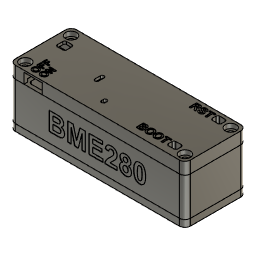
T-Go Energy Thicc v13 (Autodesk Fusion 360 design; units mm, degrees)
Autodesk Fusion 360 part; units mm, degrees
note: some values were not read from the file. Chosen so that the rebuilt part matches the saved one: which face or edge a step refers to; the layout of a text. Set by a fixed rule: which sketch regions a step uses.
(part 1 of 2)
sketch "Sketch1" plane through (0, 0, 0) normal (0, 0, 1) x (1, 0, 0)
  line L0 (0, 0) -> (91.19, 0)
  line L1 (91.19, 0) -> (91.19, -29)
  line L2 (91.19, -29) -> (0, -29)
  line L3 (0, -29) -> (0, 0)
  line L4 (89.22, -2) -> (89.22, -27) construction
  line L5 (89.22, -27) -> (1.97, -27) construction
  line L6 (1.97, -27) -> (1.97, -2) construction
  line L7 (45.595, 0) -> (45.595, -29) construction
  line L8 (0, -14.5) -> (91.19, -14.5) construction
  circle A0 centre (1.97, -2) radius 1.5
  circle A1 centre (89.22, -2) radius 1.5
  circle A2 centre (89.22, -27) radius 1.5
  circle A3 centre (1.97, -27) radius 1.5
  line L9 (7, 2) -> (15, 2)
  line L10 (15, 2) -> (15, -5)
  line L11 (15, -5) -> (7, -5)
  line L12 (7, -5) -> (7, 2)
  line L13 (3.5, -7) -> (6.5, -7)
  line L14 (6.5, -7) -> (6.5, -10)
  line L15 (6.5, -10) -> (3.5, -10)
  line L16 (3.5, -10) -> (3.5, -7)
  line L17 (6, -25.5) -> (15, -25.5)
  line L18 (15, -25.5) -> (15, -29.5)
  line L19 (15, -29.5) -> (6, -29.5)
  line L20 (6, -29.5) -> (6, -25.5)
  line L21 (9, -29.5) -> (11, -29.5)
  line L22 (11, -29.5) -> (11, -31.5)
  line L23 (11, -31.5) -> (9, -31.5)
  line L24 (9, -31.5) -> (9, -29.5)
  line L25 (80.19, 0) -> (84.19, 0)
  line L26 (84.19, 0) -> (84.19, -3)
  line L27 (84.19, -3) -> (80.19, -3)
  line L28 (80.19, -3) -> (80.19, 0)
  line L29 (80.19, -24) -> (84.19, -24)
  line L30 (84.19, -24) -> (84.19, -27)
  line L31 (84.19, -27) -> (80.19, -27)
  line L32 (80.19, -27) -> (80.19, -24)
  line L33 (29, -17) -> (31, -17)
  line L34 (31, -17) -> (31, -12)
  line L35 (31, -12) -> (29, -12)
  line L36 (29, -12) -> (29, -17)
  line L37 (41, -25.4) -> (43, -25.4)
  line L38 (43, -25.4) -> (43, -22.4)
  line L39 (43, -22.4) -> (41, -22.4)
  line L40 (41, -22.4) -> (41, -25.4)
  line L41 (1.97, -2) -> (89.22, -2) construction
  dimension "d1" = 91.19
  dimension "d2" = 29
  dimension "d3" = 3
  dimension "d4" = 84.25
  dimension "d5" = 22
  dimension "d6" = 2
  dimension "d7" = 7
  dimension "d8" = 5
  dimension "d9" = 8
  dimension "d10" = 3.5
  dimension "d11" = 7
  dimension "d12" = 3
  dimension "d13" = 3
  dimension "d14" = 6
  dimension "d15" = 9
  dimension "d16" = 0.5
  dimension "d17" = 9
  dimension "d18" = 11
  dimension "d19" = 2.5
  dimension "d20" = 3.5
  dimension "d21" = 7
  dimension "d22" = 4
  dimension "d23" = 3
  dimension "d24" = 2
  dimension "d84" = 29
  dimension "d85" = 12
  dimension "d87" = 12
  dimension "d88" = 2
  dimension "d110" = 2
  dimension "d111" = 3
  dimension "d126" = 3.6
  dimension "d127" = 41
  constraint horizontal L0
  constraint vertical L1
  constraint horizontal L2
  constraint vertical L3
  constraint coincident L0.start L3.end
  constraint vertical L4
  constraint horizontal L5
  constraint vertical L6
  constraint midpoint L0 L7.start
  constraint midpoint L2 L7.end
  constraint midpoint L3 L8.start
  constraint midpoint L1 L8.end
  constraint symmetric L4 L6 L7
  constraint coincident L6.end A0.centre
  constraint coincident L4.start A1.centre
  constraint coincident L4.end L5.start
  constraint coincident L5.end L6.start
  constraint equal A0 A3
  constraint equal A1 A3
  constraint equal A1 A2
  constraint horizontal L9
  constraint vertical L10
  constraint horizontal L11
  constraint vertical L12
  constraint horizontal L13
  constraint vertical L14
  constraint horizontal L15
  constraint vertical L16
  constraint horizontal L17
  constraint vertical L18
  constraint horizontal L19
  constraint vertical L20
  constraint horizontal L21
  constraint vertical L22
  constraint horizontal L23
  constraint vertical L24
  constraint coincident L19 L21.start
  constraint horizontal L25
  constraint vertical L26
  constraint horizontal L27
  constraint vertical L28
  constraint horizontal L29
  constraint vertical L30
  constraint horizontal L31
  constraint vertical L32
  constraint coincident L0 L25.end
  constraint collinear L26 L30
  constraint collinear L28 L32
  constraint equal L28 L32
  constraint horizontal L33
  constraint vertical L34
  constraint horizontal L35
  constraint vertical L36
  constraint horizontal L37
  constraint vertical L38
  constraint horizontal L39
  constraint vertical L40
  constraint perpendicular L4 L41
  constraint symmetric L5 L8 L41
  measures "d1" distance of L0.start L0.end
  measures "d2" distance of L0 L2
  measures "d3" diameter of A0
  measures "d4" distance of A0 A1
  measures "d5" distance of A1 A2
  measures "d6" distance of L0 L9
  measures "d7" distance of L3 L12
  measures "d8" distance of L0 L11
  measures "d9" distance of L9.start L9.end
  measures "d10" distance of L3 L16
  measures "d11" distance of L0 L13
  measures "d12" distance of L13 L15
  measures "d13" distance of L14 L16
  measures "d14" distance of L3 L20
  measures "d15" distance of L18 L20
  measures "d16" distance of L2 L19
  measures "d17" distance of L3 L24
  measures "d18" distance of L3 L22
  measures "d19" distance of L2 L23
  measures "d20" distance of L2 L17
  measures "d21" distance of L1 L26
  measures "d22" distance of L25.start L25.end
  measures "d23" distance of L25 L27
  measures "d24" distance of L2 L31
  measures "d84" distance of L3 L36
  measures "d85" distance of L0 L35
  measures "d87" distance of L2 L33
  measures "d88" distance of L34 L36
  measures "d110" distance of L38 L40
  measures "d111" distance of L37.end L38.end
  measures "d126" distance of L2 L37
  measures "d127" distance of L3 L40
sketch "Sketch2" plane through (0, 0, 0) normal (0, 0, 1) x (1, 0, 0)
  line L0 (0, 0) -> (91.19, 0)
  line L1 (0, -29) -> (0, 0)
  line L2 (91.19, 0) -> (91.19, -29)
  line L3 (91.19, -29) -> (0, -29)
  line L4 (7, -4) -> (84.19, -4)
  line L5 (84.19, -4) -> (84.19, -25)
  line L6 (84.19, -25) -> (7, -25)
  line L7 (7, -25) -> (7, -4)
  line L8 (0, -14.5) -> (91.19, -14.5) construction
  line L9 (45.595, 0) -> (45.595, -29) construction
  line L10 (84.19, -10.5) -> (90.19, -10.5)
  line L11 (90.19, -10.5) -> (90.19, -18.5)
  line L12 (90.19, -18.5) -> (84.19, -18.5)
  line L13 (84.19, -18.5) -> (84.19, -10.5)
  line L14 (7, -10.5) -> (1, -10.5)
  line L15 (1, -10.5) -> (1, -18.5)
  line L16 (1, -18.5) -> (7, -18.5)
  line L17 (7, -18.5) -> (7, -10.5)
  line L18 (6, -29.5) -> (6, -25.5) construction
  line L19 (15, -25.5) -> (15, -29.5) construction
  line L20 (6, -27.5) -> (15, -27.5) construction
  circle A0 centre (10.5, -27.5) radius 0.75
  circle A1 centre (13, -27.5) radius 0.75
  circle A2 centre (8, -27.5) radius 0.75
  line L21 (10.5, -27.5) -> (10.5, -21.4329) construction
  dimension "d25" = 7
  dimension "d26" = 4
  dimension "d27" = 1
  dimension "d28" = 8
  dimension "d29" = 1.5
  dimension "d30" = 5
  dimension "d31" = 1.5
  constraint horizontal L4
  constraint vertical L5
  constraint horizontal L6
  constraint vertical L7
  constraint midpoint L1 L8.start
  constraint midpoint L2 L8.end
  constraint symmetric L4 L6 L8
  constraint midpoint L0 L9.start
  constraint midpoint L3 L9.end
  constraint symmetric L5 L7 L9
  constraint horizontal L10
  constraint vertical L11
  constraint horizontal L12
  constraint vertical L13
  constraint coincident L5 L10.start
  constraint horizontal L14
  constraint vertical L15
  constraint horizontal L16
  constraint vertical L17
  constraint coincident L7 L14.start
  constraint symmetric L8 L14 L16
  constraint symmetric L8 L10 L12
  constraint equal L10 L14
  constraint midpoint L18 L20.start
  constraint midpoint L19 L20.end
  constraint midpoint L20 A0.centre
  constraint coincident L20 A1.centre
  constraint coincident L20 A2.centre
  constraint coincident A0.centre L21.start
  constraint perpendicular L20 L21
  constraint symmetric A1 A2 L21
  constraint collinear L10 L14
  measures "d25" distance of L1 L7
  measures "d26" distance of L0 L4
  measures "d27" distance of L2 L11
  measures "d28" distance of L10 L12
  measures "d29" diameter of A0
  measures "d30" distance of A1.centre A2.centre
  measures "d31" diameter of A2
sketch "Sketch3" plane through (0, 0, 0) normal (0, 0, 1) x (1, 0, 0)
  circle A0 centre (1.97, -2) radius 1.5
  circle A1 centre (1.97, -27) radius 1.5
  circle A2 centre (89.22, -2) radius 1.5
  circle A3 centre (89.22, -27) radius 1.5
  line L0 (7, -5) -> (7, 2)
  line L1 (15, 2) -> (15, -5)
  line L2 (15, -5) -> (7, -5)
  line L3 (7, 2) -> (15, 2)
  line L4 (6, -29.5) -> (6, -25.5)
  line L5 (6, -25.5) -> (15, -25.5)
  line L6 (15, -25.5) -> (15, -29.5)
  line L7 (15.5, 2) -> (15.5, -5.5)
  line L8 (15.5, -5.5) -> (6.5, -5.5)
  line L9 (6.5, -5.5) -> (6.5, 2)
  line L10 (5.5, -29.5) -> (5.5, -25)
  line L11 (5.5, -25) -> (15.5, -25)
  line L12 (15.5, -25) -> (15.5, -29.5)
  line L13 (80.19, -3) -> (80.19, 0)
  line L14 (84.19, 0) -> (84.19, -3)
  line L15 (84.19, -3) -> (80.19, -3)
  line L16 (80.19, -27) -> (80.19, -24)
  line L17 (80.19, -24) -> (84.19, -24)
  line L18 (84.19, -24) -> (84.19, -27)
  line L19 (84.19, -27) -> (80.19, -27)
  line L20 (79.69, -27.5) -> (79.69, -23.5)
  line L21 (79.69, -23.5) -> (84.69, -23.5)
  line L22 (84.69, -23.5) -> (84.69, -27.5)
  line L23 (84.69, -27.5) -> (79.69, -27.5)
  line L24 (0, 0) -> (91.19, 0)
  line L25 (91.19, 0) -> (91.19, -29)
  line L26 (91.19, -29) -> (0, -29)
  line L27 (0, -29) -> (0, 0)
  line L28 (-2.25, 2.25) -> (93.44, 2.25)
  line L29 (93.44, 2.25) -> (93.44, -31.25)
  line L30 (93.44, -31.25) -> (-2.25, -31.25)
  line L31 (-2.25, -31.25) -> (-2.25, 2.25)
  line L32 (78.19, 0) -> (78.19, -29)
  line L33 (79.69, -3.5) -> (78.19, -3.5)
  line L34 (7, -25) -> (7, -14)
  line L35 (7, -14) -> (0, -14)
  line L36 (6.5, -5.5) -> (0, -5.5)
  line L37 (6.5, 2) -> (6.5, 2.25)
  line L38 (15.5, 2) -> (15.5, 2.25)
  line L39 (5.5, -29.5) -> (5.5, -31.25)
  line L40 (15.5, -29.5) -> (15.5, -31.25)
  line L41 (80.19, 0) -> (84.19, 0)
  line L42 (84.69, -3.5) -> (79.69, -3.5)
  line L43 (79.69, -3.5) -> (79.69, 0.5)
  line L44 (79.69, 0.5) -> (84.69, 0.5)
  line L45 (84.69, 0.5) -> (84.69, -3.5)
  circle A4 centre (1.97, -2) radius 1.625
  circle A5 centre (89.22, -2) radius 1.625
  circle A6 centre (89.22, -27) radius 1.625
  circle A7 centre (1.97, -27) radius 1.625
  dimension "d32" = -0.5
  dimension "d33" = -0.5
  dimension "d35" = -0.5
  dimension "d36" = -2.25
  dimension "d39" = 13
  dimension "d40" = 7
  dimension "d41" = 15
  dimension "d49" = -0.5
  dimension "d128" = 3.25
  constraint coincident L24 L32.start
  constraint coincident L26 L32.end
  constraint perpendicular L26 L32
  constraint coincident L32 L33.end
  constraint perpendicular L32 L33
  constraint perpendicular L11 L34
  constraint coincident L27 L35.end
  constraint perpendicular L27 L35
  constraint coincident L11 L34.start
  constraint coincident L27 L36.end
  constraint perpendicular L27 L36
  constraint coincident L28 L37.end
  constraint perpendicular L28 L37
  constraint coincident L28 L38.end
  constraint perpendicular L28 L38
  constraint coincident L30 L39.end
  constraint perpendicular L30 L39
  constraint coincident L30 L40.end
  constraint perpendicular L30 L40
  constraint coincident L33.start L42.end
  constraint concentric A0 A4
  constraint concentric A2 A5
  constraint concentric A3 A6
  constraint concentric A1 A7
  constraint equal A4 A5
  constraint equal A5 A6
  constraint equal A6 A7
  measures "d39" distance of L25 L32
  measures "d40" distance of L27 L34
  measures "d41" distance of L26 L35
  measures "d128" diameter of A4
extrude "Extrude1" add sketch "Sketch1" sketch "Sketch3" along normal blind 5 contours L0 L10 L11 L12 of sketch 2 contours L0 L1 L2 L7 L8 L9 L24 | L0 L1 L3 L7 L9 L24 L28 L37 L38 | L0 L1 L3 L24 | L9 L10 L24 L26 L27 L28 L30 L31 L37 L39 | L9 L24 L27 L36 | L7 L8 L11 L12 L24 L26 L27 L32 L34 L35 L36 | L7 L12 L24 L25 L26 L28 L29 L30 L38 L40 L43 L44 L45 | L24 L32 L33 L43 | L10 L11 L26 L27 L34 L35 | L24 L25 L26 L32 L33 L42 L45 | L10 L12 L26 L30 L39 L40 | L4 L5 L6 L10 L11 L12 L26 | L4 L5 L6 L26 makes body 1
extrude "Extrude2" cut sketch "Sketch3" along normal blind 3.5 contours L7 L8 L11 L12 L24 L26 L27 L32 L34 L35 L36 bodies 1
extrude "Extrude3" cut sketch "Sketch3" along normal blind 4 contours L10 L12 L26 L30 L39 L40 | L4 L5 L6 L10 L11 L12 L26 | L4 L5 L6 L26 bodies 1
extrude "Extrude4" cut sketch "Sketch3" along normal blind 4 contours L0 L1 L2 L7 L8 L9 L24 | L0 L1 L2 L24 | L0 L1 L3 L7 L9 L24 L28 L37 L38 | L0 L1 L3 L24 bodies 1
fillet "Fillet1" radius 3 4 edges at (93.44, -31.25, 2.5) (93.44, 2.25, 2.5) (-2.25, 2.25, 2.5) (-2.25, -31.25, 2.5) on bodies 1
sketch "Sketch4" plane through (0, 0, 0) normal (0, 0, -1) x (1, 0, 0)
  arc A0 (0.75, 31.25) -> (-2.25, 28.25) centre (0.75, 28.25) ccw
  line L0 (-2.25, 28.25) -> (-2.25, 0.75)
  arc A1 (-2.25, 0.75) -> (0.75, -2.25) centre (0.75, 0.75) ccw
  line L1 (0.75, -2.25) -> (6.5, -2.25)
  line L2 (6.5, -2.25) -> (6.5, 5.5)
  line L3 (6.5, 5.5) -> (0, 5.5)
  line L4 (0, 5.5) -> (0, 14)
  line L5 (0, 14) -> (7, 14)
  line L6 (7, 14) -> (7, 25)
  line L7 (7, 25) -> (5.5, 25)
  line L8 (5.5, 25) -> (5.5, 31.25)
  line L9 (5.5, 31.25) -> (0.75, 31.25)
  line L10 (91.19, 29) -> (0, 29)
  line L11 (0, 29) -> (0, 0)
  line L12 (0, 0) -> (91.19, 0)
  line L13 (91.19, 0) -> (91.19, 29)
  arc A2 (90.44, -2.25) -> (93.44, 0.75) centre (90.44, 0.75) ccw
  line L14 (93.44, 0.75) -> (93.44, 28.25)
  arc A3 (93.44, 28.25) -> (90.44, 31.25) centre (90.44, 28.25) ccw
  line L15 (90.44, 31.25) -> (15.5, 31.25)
  line L16 (15.5, 31.25) -> (15.5, 29)
  line L17 (15.5, 29) -> (78.19, 29)
  line L18 (78.19, 29) -> (78.19, 0)
  line L19 (78.19, 0) -> (15.5, 0)
  line L20 (15.5, 0) -> (15.5, -2.25)
  line L21 (15.5, -2.25) -> (90.44, -2.25)
  line L22 (84.69, -0.5) -> (79.69, -0.5)
  line L23 (79.69, -0.5) -> (79.69, 3.5)
  line L24 (79.69, 3.5) -> (84.69, 3.5)
  line L25 (84.69, 3.5) -> (84.69, -0.5)
  line L26 (84.69, 27.5) -> (84.69, 23.5)
  line L27 (84.69, 23.5) -> (79.69, 23.5)
  line L28 (79.69, 23.5) -> (79.69, 27.5)
  line L29 (79.69, 27.5) -> (84.69, 27.5)
  circle A4 centre (1.97, 27) radius 1.625
  circle A5 centre (1.97, 2) radius 1.625
  circle A6 centre (89.22, 27) radius 1.625
  circle A7 centre (89.22, 2) radius 1.625
extrude "Extrude5" add sketch "Sketch4" along normal blind 1.6 contours A0 L0 A1 L1 L2 L4 L8 L9 L10 L11 L12 | L10 L12 L13 A2 L14 A3 L15 L16 L17 L19 L20 L21 L22 L23 L25 bodies 1
move_face "OffsetFaces1" offset -0.25 7 faces at (36.3967, -29, 0.6333) (3.6667, -29, -0.5333) (0, -11.1667, 1.1667) (2.1667, 0, -0.5333) (36.3967, 0, 0.6333) (91.19, -9.6667, -0.5333) (86.8567, 0, -0.5333) on bodies 1
fillet "Fillet2" radius 1 4 edges at (-0.25, 0.25, -0.8) (-0.25, -29.25, -0.8) (91.44, -29.25, -0.8) (91.44, 0.25, -0.8) on bodies 1
sketch "Sketch5" plane through (0, 0, 5) normal (0, 0, 1) x (-1, 0, 0)
  arc A0 (2.25, 28.25) -> (-0.75, 31.25) centre (-0.75, 28.25) ccw
  line L0 (-0.75, 31.25) -> (-90.44, 31.25)
  arc A1 (-90.44, 31.25) -> (-93.44, 28.25) centre (-90.44, 28.25) ccw
  line L1 (-93.44, 28.25) -> (-93.44, 0.75)
  arc A2 (-93.44, 0.75) -> (-90.44, -2.25) centre (-90.44, 0.75) ccw
  line L2 (-90.44, -2.25) -> (-0.75, -2.25)
  arc A3 (-0.75, -2.25) -> (2.25, 0.75) centre (-0.75, 0.75) ccw
  line L3 (2.25, 0.75) -> (2.25, 28.25)
  line L4 (-84.69, 23.5) -> (-84.69, 27.5)
  line L5 (-84.69, 27.5) -> (-79.69, 27.5)
  line L6 (-79.69, 27.5) -> (-79.69, 23.5)
  line L7 (-79.69, 23.5) -> (-84.69, 23.5)
  line L8 (-79.69, -0.5) -> (-84.69, -0.5)
  line L9 (-84.69, -0.5) -> (-84.69, 3.5)
  line L10 (-84.69, 3.5) -> (-79.69, 3.5)
  line L11 (-79.69, 3.5) -> (-79.69, -0.5)
  line L12 (-3.5, 7) -> (-6.5, 7)
  line L13 (-3.5, 10) -> (-3.5, 7)
  line L14 (-6.5, 10) -> (-3.5, 10)
  line L15 (-6.5, 7) -> (-6.5, 10)
  line L16 (-2.5, 11) -> (-2.5, 6)
  line L17 (-2.5, 6) -> (-7.5, 6)
  line L18 (-7.5, 6) -> (-7.5, 11)
  line L19 (-7.5, 11) -> (-2.5, 11)
  circle A4 centre (-1.97, 2) radius 1.625
  circle A5 centre (-89.22, 2) radius 1.625
  circle A6 centre (-89.22, 27) radius 1.625
  circle A7 centre (-1.97, 27) radius 1.625
  dimension "d56" = -1
extrude "Extrude6" cut sketch "Sketch5" against normal blind 18 contours L12 L13 L14 L15 | L16 L17 L18 L19 bodies 1
sketch "Sketch6" plane through (-2.25, 0, 0) normal (-1, 0, 0) x (0, -1, 0)
  line L0 (28.25, -1.6) -> (28.25, 5)
  line L1 (28.25, 5) -> (0.75, 5)
  line L2 (0.75, 5) -> (0.75, -1.6)
  line L3 (0.75, -1.6) -> (28.25, -1.6)
  line L4 (6, 3.5) -> (11, 3.5)
  line L5 (11, 3.5) -> (11, 5)
  line L6 (11, 5) -> (6, 5)
  line L7 (6, 5) -> (6, 3.5)
  line L8 (29, 0) -> (0, 0)
  line L9 (6, 3.5) -> (11, 3.5)
  line L10 (11, 3.5) -> (11, 0)
  line L11 (11, 0) -> (6, 0)
  line L12 (6, 0) -> (6, 3.5)
  constraint horizontal L9
  constraint vertical L10
  constraint horizontal L11
  constraint vertical L12
  constraint coincident L8 L10.end
  constraint coincident L4.start L7.end
  constraint coincident L4.end L5.start
extrude "Extrude7" cut sketch "Sketch6" against normal blind 8.5 contours L4 L8 L9 L10 L11 L12 bodies 1
fillet "Fillet3" radius 1 8 edges at (7.5, -6, 4.25) (2.5, -6, 4.25) (2.5, -11, 4.25) (7.5, -11, 4.25) (-1.25, -11, 0) (-1.25, -6, 0) (-1.25, -6, 3.5) (-1.25, -11, 3.5) on bodies 1
extrude "Extrude12" cut sketch "Sketch1" along normal blind 14 contours L33 L34 L35 L36 | L37 L38 L39 L40 bodies 1
fillet "Fillet5" radius 1 8 edges at (29, -12, 4.25) (31, -12, 4.25) (31, -17, 4.25) (29, -17, 4.25) (43, -25.4, 4.25) (41, -25.4, 4.25) (41, -22.4, 4.25) (43, -22.4, 4.25) on bodies 1
sketch "Sketch8" plane through (0, 0, -1.6) normal (0, 0, -1) x (1, 0, 0)
  line L0 (84.69, -0.5) -> (79.69, -0.5)
  line L1 (79.69, -0.5) -> (79.69, -0.25)
  line L2 (79.69, -0.25) -> (15.5, -0.25)
  line L3 (15.5, -0.25) -> (15.5, -2.25)
  line L4 (15.5, -2.25) -> (90.44, -2.25)
  arc A0 (90.44, -2.25) -> (93.44, 0.75) centre (90.44, 0.75) ccw
  line L5 (93.44, 0.75) -> (93.44, 28.25)
  arc A1 (93.44, 28.25) -> (90.44, 31.25) centre (90.44, 28.25) ccw
  line L6 (90.44, 31.25) -> (15.5, 31.25)
  line L7 (15.5, 31.25) -> (15.5, 29.25)
  line L8 (15.5, 29.25) -> (90.44, 29.25)
  arc A2 (91.44, 28.25) -> (90.44, 29.25) centre (90.44, 28.25) ccw
  line L9 (91.44, 28.25) -> (91.44, 0.75)
  arc A3 (90.44, -0.25) -> (91.44, 0.75) centre (90.44, 0.75) ccw
  line L10 (90.44, -0.25) -> (84.69, -0.25)
  line L11 (84.69, -0.25) -> (84.69, -0.5)
  arc A4 (0.75, 31.25) -> (-2.25, 28.25) centre (0.75, 28.25) ccw
  line L12 (5.5, 31.25) -> (0.75, 31.25)
  line L13 (5.5, 31.25) -> (15.5, 31.25)
  line L14 (90.44, 31.25) -> (15.5, 31.25)
  arc A5 (93.44, 28.25) -> (90.44, 31.25) centre (90.44, 28.25) ccw
  line L15 (93.44, 0.75) -> (93.44, 28.25)
  arc A6 (90.44, -2.25) -> (93.44, 0.75) centre (90.44, 0.75) ccw
  line L16 (15.5, -2.25) -> (90.44, -2.25)
  line L17 (15.5, -2.25) -> (6.5, -2.25)
  line L18 (0.75, -2.25) -> (6.5, -2.25)
  arc A7 (-2.25, 0.75) -> (0.75, -2.25) centre (0.75, 0.75) ccw
  line L19 (-2.25, 28.25) -> (-2.25, 0.75)
  line L20 (1, 18.5) -> (7, 18.5)
  line L21 (1, 10.5) -> (1, 18.5)
  line L22 (7, 10.5) -> (1, 10.5)
  line L23 (84.19, 25) -> (7, 25)
  line L24 (84.19, 4) -> (84.19, 25)
  line L25 (90.19, 18.5) -> (84.19, 18.5)
  line L26 (90.19, 10.5) -> (90.19, 18.5)
  line L27 (84.19, 10.5) -> (90.19, 10.5)
  line L28 (7, 4) -> (84.19, 4)
  line L29 (7, 25) -> (7, 4)
  circle A8 centre (8, 27.5) radius 0.75 construction
  circle A9 centre (10.5, 27.5) radius 0.75 construction
  circle A10 centre (13, 27.5) radius 0.75 construction
  circle A11 centre (1.97, 27) radius 1.5 construction
  circle A12 centre (89.22, 27) radius 1.5 construction
  circle A13 centre (89.22, 2) radius 1.5 construction
  circle A14 centre (1.97, 2) radius 1.5 construction
  circle A15 centre (1.97, 27) radius 1.4
  circle A16 centre (89.22, 27) radius 1.4
  circle A17 centre (89.22, 2) radius 1.4
  circle A18 centre (1.97, 2) radius 1.4
  line L30 (71.19, 31.25) -> (71.19, 25)
  line L31 (0, 29) -> (0, 0) construction
  line L32 (91.19, 29) -> (0, 29) construction
  line L33 (0, 0) -> (91.19, 0) construction
  line L34 (91.19, 0) -> (91.19, 29) construction
  line L35 (71.19, 4) -> (71.19, -2.25)
  line L36 (16.75, 4) -> (16.75, -2.25)
  line L37 (7, 25) -> (7, 31.25)
  line L38 (15.5, 29.25) -> (90.44, 29.25)
  line L39 (79.69, -0.25) -> (15.5, -0.25)
  line L40 (15.5, 29.25) -> (7, 29.25)
  line L41 (6.5, 7) -> (6.5, 10)
  line L42 (3.5, 7) -> (6.5, 7)
  line L43 (3.5, 10) -> (3.5, 7)
  line L44 (6.5, 10) -> (3.5, 10)
  dimension "d72" = 2.8
  dimension "d73" = 20
  dimension "d74" = 19
  constraint concentric A11 A15
  constraint concentric A12 A16
  constraint concentric A13 A17
  constraint concentric A14 A18
  constraint equal A15 A18
  constraint equal A15 A16
  constraint equal A16 A17
  constraint coincident L14 L30.start
  constraint perpendicular L8 L30
  constraint coincident L23 L30.end
  constraint coincident L28 L35.start
  constraint coincident L16 L35.end
  constraint perpendicular L16 L35
  constraint collinear L30 L35
  constraint coincident L28 L36.start
  constraint coincident L4 L36.end
  constraint perpendicular L4 L36
  constraint coincident L23.end L29.start
  constraint perpendicular L23 L37
  constraint coincident L13 L37.end
  constraint coincident L7.end L8.start
  constraint coincident L37 L40.end
  constraint perpendicular L37 L40
  measures "d72" diameter of A15
  measures "d73" distance of L30 L34
  measures "d74" distance of L19 L36
extrude "Extrude9" add sketch "Sketch8" along normal blind 21 separate body contours L0 L1 L2 L4 A0 L5 A1 L6 L8 A2 L9 A3 L10 L11 L14 A5 L15 A6 L16 L30 L35 L38 L39 | L0 L1 L2 L8 A2 L9 A3 L10 L11 L23 L24 L25 L26 L27 L28 L30 L35 L38 L39 | L2 L4 L16 L35 L36 L39 | L2 L3 L4 L16 L36 L39 | L2 L3 A4 L12 L13 L17 L18 A7 L19 L20 L21 L22 L28 L29 L36 L37 L39 | L6 L7 L8 L14 L30 L38 | L7 L13 L37 L40 | L41 L42 L43 L44 makes body 2
sketch "Sketch9" plane through (0, 0, -22.6) normal (0, 0, -1) x (1, 0, 0)
  line L0 (7, 29.25) -> (71.19, 29.25)
  line L1 (71.19, 29.25) -> (71.19, 25)
  line L2 (71.19, 25) -> (84.19, 25)
  line L3 (84.19, 25) -> (84.19, 18.5)
  line L4 (84.19, 18.5) -> (90.19, 18.5)
  line L5 (90.19, 18.5) -> (90.19, 10.5)
  line L6 (90.19, 10.5) -> (84.19, 10.5)
  line L7 (84.19, 10.5) -> (84.19, 4)
  line L8 (84.19, 4) -> (71.19, 4)
  line L9 (71.19, 4) -> (71.19, -0.25)
  line L10 (71.19, -0.25) -> (16.75, -0.25)
  line L11 (16.75, -0.25) -> (16.75, 4)
  line L12 (16.75, 4) -> (7, 4)
  line L13 (7, 4) -> (7, 10.5)
  line L14 (7, 10.5) -> (1, 10.5)
  line L15 (1, 10.5) -> (1, 18.5)
  line L16 (1, 18.5) -> (7, 18.5)
  line L17 (7, 18.5) -> (7, 29.25)
  circle A0 centre (1.97, 27) radius 1.4
  circle A1 centre (89.22, 27) radius 1.4
  circle A2 centre (89.22, 2) radius 1.4
  circle A3 centre (1.97, 2) radius 1.4
  line L18 (90.44, 31.25) -> (0.75, 31.25)
  arc A4 (0.75, 31.25) -> (-2.25, 28.25) centre (0.75, 28.25) ccw
  line L19 (-2.25, 28.25) -> (-2.25, 0.75)
  arc A5 (-2.25, 0.75) -> (0.75, -2.25) centre (0.75, 0.75) ccw
  line L20 (0.75, -2.25) -> (90.44, -2.25)
  arc A6 (90.44, -2.25) -> (93.44, 0.75) centre (90.44, 0.75) ccw
  line L21 (93.44, 0.75) -> (93.44, 28.25)
  arc A7 (93.44, 28.25) -> (90.44, 31.25) centre (90.44, 28.25) ccw
  line L22 (7, 18.5) -> (7, 10.5)
  line L23 (84.19, 18.5) -> (84.19, 10.5)
  circle A8 centre (13, 27.5) radius 0.75 construction
  circle A9 centre (10.5, 27.5) radius 0.75 construction
  circle A10 centre (8, 27.5) radius 0.75 construction
  line L24 (16.75, 4) -> (71.19, 4)
  line L25 (71.19, 25) -> (7, 25)
  point P0 (8, 27.5)
  point P1 (10.5, 27.5)
  constraint coincident L16.end L17.start
  constraint coincident L13.end L14.start
  constraint coincident L3.end L4.start
  constraint coincident L6.end L7.start
  constraint coincident L11.end L12.start
  constraint coincident L8.end L9.start
  constraint coincident L1.end L2.start
  constraint coincident L17 L25.end
  constraint perpendicular L17 L25
extrude "Extrude10" add sketch "Sketch9" against normal blind 18 contours L14 L15 L16 L22 | L4 L5 L6 L23 bodies 2
extrude "Extrude11" add sketch "Sketch9" against normal blind 2.5 contours L0 L1 L17 L25 | L9 L10 L11 L24 bodies 2
sketch "Sketch10" plane through (0, 0, -1.6) normal (0, 0, 1) x (-1, 0, 0)
  line L0 (-71.19, 29.25) -> (-7, 29.25)
  line L1 (-7, 29.25) -> (-7, 18.5)
  line L2 (-7, 18.5) -> (-1, 18.5)
  line L3 (-1, 18.5) -> (-1, 10.5)
  line L4 (-1, 10.5) -> (-7, 10.5)
  line L5 (-7, 10.5) -> (-7, 4)
  line L6 (-7, 4) -> (-16.75, 4)
  line L7 (-16.75, 4) -> (-16.75, -0.25)
  line L8 (-16.75, -0.25) -> (-71.19, -0.25)
  line L9 (-71.19, -0.25) -> (-71.19, 4)
  line L10 (-71.19, 4) -> (-84.19, 4)
  line L11 (-84.19, 4) -> (-84.19, 10.5)
  line L12 (-84.19, 10.5) -> (-90.19, 10.5)
  line L13 (-90.19, 10.5) -> (-90.19, 18.5)
  line L14 (-90.19, 18.5) -> (-84.19, 18.5)
  line L15 (-84.19, 18.5) -> (-84.19, 25)
  circle A0 centre (-1.97, 2) radius 1.4
  circle A1 centre (-1.97, 27) radius 1.4
  circle A2 centre (-89.22, 2) radius 1.4
  line L16 (-0.75, 31.25) -> (-90.44, 31.25)
  line L17 (-93.44, 28.25) -> (-93.44, 0.75)
  arc A3 (-93.44, 0.75) -> (-90.44, -2.25) centre (-90.44, 0.75) ccw
  line L18 (-90.44, -2.25) -> (-0.75, -2.25)
  arc A4 (-0.75, -2.25) -> (2.25, 0.75) centre (-0.75, 0.75) ccw
  line L19 (2.25, 0.75) -> (2.25, 28.25)
  arc A5 (2.25, 28.25) -> (-0.75, 31.25) centre (-0.75, 28.25) ccw
  line L20 (-91.19, 29) -> (0, 29)
  line L21 (-91.19, 0) -> (-91.19, 29)
  line L22 (-71.19, 25) -> (-7, 25)
  line L23 (-71.19, 25) -> (-84.19, 25)
  line L24 (-71.69, 25) -> (-61.19, 25)
  line L25 (-61.19, 25) -> (-61.19, 30)
  line L26 (-61.19, 30) -> (-71.69, 30)
  line L27 (-71.69, 30) -> (-71.69, 25)
  dimension "d94" = 19.5
  dimension "d95" = 1
  dimension "d96" = 30
  constraint horizontal L24
  constraint vertical L25
  constraint horizontal L26
  constraint vertical L27
  constraint coincident L22 L24.start
  measures "d94" distance of L21 L27
  measures "d95" distance of L20 L26
  measures "d96" distance of L21 L25
extrude "Extrude13" cut sketch "Sketch10" against normal blind 29 contours L20 L25 L26 L27 | L20 L22 L23 L24 L25 L27 bodies 2
sketch "Sketch11" plane through (0, 0, 5) normal (0, 0, 1) x (-1, 0, 0)
  line L0 (-31, 13) -> (-31, 16)
  arc A0 (-29, 16) -> (-31, 16) centre (-30, 16) ccw
  line L1 (-29, 16) -> (-29, 13)
  arc A1 (-31, 13) -> (-29, 13) centre (-30, 13) ccw
  line L2 (-3.5, 6) -> (-6.5, 6)
  arc A2 (-7.5, 7) -> (-6.5, 6) centre (-6.5, 7) ccw
  line L3 (-7.5, 7) -> (-7.5, 10)
  arc A3 (-6.5, 11) -> (-7.5, 10) centre (-6.5, 10) ccw
  line L4 (-6.5, 11) -> (-3.5, 11)
  arc A4 (-2.5, 10) -> (-3.5, 11) centre (-3.5, 10) ccw
  line L5 (-2.5, 10) -> (-2.5, 7)
  arc A5 (-3.5, 6) -> (-2.5, 7) centre (-3.5, 7) ccw
  arc A6 (2.25, 28.25) -> (-0.75, 31.25) centre (-0.75, 28.25) ccw
  line L6 (-0.75, 31.25) -> (-90.44, 31.25)
  arc A7 (-90.44, 31.25) -> (-93.44, 28.25) centre (-90.44, 28.25) ccw
  line L7 (-93.44, 28.25) -> (-93.44, 0.75)
  arc A8 (-93.44, 0.75) -> (-90.44, -2.25) centre (-90.44, 0.75) ccw
  line L8 (-90.44, -2.25) -> (-0.75, -2.25)
  arc A9 (-0.75, -2.25) -> (2.25, 0.75) centre (-0.75, 0.75) ccw
  line L9 (2.25, 0.75) -> (2.25, 28.25)
  line L10 (-84.69, 23.5) -> (-84.69, 27.5)
  line L11 (-84.69, 27.5) -> (-79.69, 27.5)
  line L12 (-79.69, 27.5) -> (-79.69, 23.5)
  line L13 (-79.69, 23.5) -> (-84.69, 23.5)
  line L14 (-79.69, -0.5) -> (-84.69, -0.5)
  line L15 (-84.69, -0.5) -> (-84.69, 3.5)
  line L16 (-84.69, 3.5) -> (-79.69, 3.5)
  line L17 (-79.69, 3.5) -> (-79.69, -0.5)
  circle A10 centre (-1.97, 2) radius 3
  circle A11 centre (-1.97, 27) radius 3
  circle A12 centre (-89.22, 2) radius 3
  circle A13 centre (-89.22, 27) radius 3
  line L18 (-43, 23.4) -> (-43, 24.4)
  arc A14 (-41, 24.4) -> (-43, 24.4) centre (-42, 24.4) ccw
  line L19 (-41, 24.4) -> (-41, 23.4)
  arc A15 (-43, 23.4) -> (-41, 23.4) centre (-42, 23.4) ccw
  circle A16 centre (-1.97, 2) radius 1.625
  circle A17 centre (-89.22, 2) radius 1.625
  circle A18 centre (-89.22, 27) radius 1.625
  circle A19 centre (-1.97, 27) radius 1.625
  dimension "d99" = 6
  constraint equal A11 A13
  constraint equal A10 A11
  constraint equal A10 A12
  measures "d99" diameter of A10
extrude "Extrude14" cut sketch "Sketch11" against normal blind 2.5 contours A10 | A11 | A12 | A13 | A16 | A17 | A18 | A19 bodies 1
move_face "OffsetFaces3" offset -1 4 faces at (7, -13.1667, -15.7667) (84.19, -13.1667, -16.6) (79.8567, -4, -14.7667) (80.0233, -25, -15.6) on bodies 2
sketch "Sketch12" plane through (0, 0, 5) normal (0, 0, 1) x (-1, 0, 0)
  circle A0 centre (-1.97, 27) radius 3
  circle A1 centre (-89.22, 2) radius 3
  circle A2 centre (-1.97, 2) radius 3
  circle A3 centre (-89.22, 27) radius 3
  line L0 (-31, 13) -> (-31, 16)
  arc A4 (-29, 16) -> (-31, 16) centre (-30, 16) ccw
  line L1 (-29, 16) -> (-29, 13)
  arc A5 (-31, 13) -> (-29, 13) centre (-30, 13) ccw
  line L2 (-3.5, 6) -> (-6.5, 6)
  arc A6 (-7.5, 7) -> (-6.5, 6) centre (-6.5, 7) ccw
  line L3 (-7.5, 7) -> (-7.5, 10)
  arc A7 (-6.5, 11) -> (-7.5, 10) centre (-6.5, 10) ccw
  line L4 (-6.5, 11) -> (-3.5, 11)
  arc A8 (-2.5, 10) -> (-3.5, 11) centre (-3.5, 10) ccw
  line L5 (-2.5, 10) -> (-2.5, 7)
  arc A9 (-3.5, 6) -> (-2.5, 7) centre (-3.5, 7) ccw
  arc A10 (2.25, 28.25) -> (-0.75, 31.25) centre (-0.75, 28.25) ccw
  line L6 (-0.75, 31.25) -> (-90.44, 31.25)
  arc A11 (-90.44, 31.25) -> (-93.44, 28.25) centre (-90.44, 28.25) ccw
  line L7 (-93.44, 28.25) -> (-93.44, 0.75)
  arc A12 (-93.44, 0.75) -> (-90.44, -2.25) centre (-90.44, 0.75) ccw
  line L8 (-90.44, -2.25) -> (-0.75, -2.25)
  arc A13 (-0.75, -2.25) -> (2.25, 0.75) centre (-0.75, 0.75) ccw
  line L9 (2.25, 0.75) -> (2.25, 28.25)
  line L10 (-43, 23.4) -> (-43, 24.4)
  arc A14 (-41, 24.4) -> (-43, 24.4) centre (-42, 24.4) ccw
  line L11 (-41, 24.4) -> (-41, 23.4)
  arc A15 (-43, 23.4) -> (-41, 23.4) centre (-42, 23.4) ccw
  line L12 (-10, 29.25) -> (-10, 12.6615) construction
  line L13 (-10, 12.6615) -> (-6.5, 12.6615) construction
  line L14 (-6.5, 12.6615) -> (-6.5, 29.25) construction
  line L15 (-6.5, 29.25) -> (-10, 29.25) construction
  line L16 (-14.5, 29.25) -> (-14.5, 7.2393) construction
  line L17 (-14.5, 7.2393) -> (-11, 7.2393) construction
  line L18 (-11, 7.2393) -> (-11, 29.25) construction
  line L19 (-11, 29.25) -> (-14.5, 29.25) construction
  line L20 (-5.5, 31.25) -> (-5.5, 25) construction
  line L21 (-5.5, 25) -> (-15.5, 25) construction
  line L22 (-15.5, 25) -> (-15.5, 31.25) construction
  line L23 (-15.5, 31.25) -> (-5.5, 31.25) construction
  line L24 (-56.9353, 9.7291) -> (-78.69, 9.7291) construction
  line L25 (-78.69, 9.7291) -> (-78.69, -0.5) construction
  line L26 (-78.69, -0.5) -> (-56.9353, -0.5) construction
  line L27 (-56.9353, -0.5) -> (-56.9353, 9.7291) construction
  line L28 (-79.69, -0.5) -> (-84.69, -0.5)
  line L29 (-59.4279, 27.5) -> (-78.69, 27.5) construction
  line L30 (-78.69, 27.5) -> (-78.69, 16.8193) construction
  line L31 (-78.69, 16.8193) -> (-59.4279, 16.8193) construction
  line L32 (-59.4279, 16.8193) -> (-59.4279, 27.5) construction
  line L33 (-84.69, 27.5) -> (-79.69, 27.5)
  dimension "d113" = 3.5
  dimension "d114" = 3.5
  dimension "d115" = 1
  dimension "d117" = 2
  dimension "d118" = 1
  dimension "d161" = 1
  text T0 "OFF" font "Arial" height 3.5 bold align left top in box 16.5885 x 3.5 at (-10, 29.25) x (0, -1) y (1, 0) spacing 1
  text T1 "ON" font "Arial" height 3.5 bold align left top in box 22.0107 x 3.5 at (-14.5, 29.25) x (0, -1) y (1, 0) spacing 1
  text T2 "RST" font "Arial" height 4 bold align right top in box 21.7547 x 10.2291 at (-56.9353, 9.7291) x (-1, 0) y (0, -1) spacing 1
  text T3 "BOOT" font "Arial" height 4 bold align right bottom in box 19.2621 x 10.6807 at (-59.4279, 27.5) x (-1, 0) y (0, -1) spacing 1
  constraint collinear L15 L19
  constraint collinear L26 L28
  constraint collinear L25 L30
  constraint collinear L29 L33
  measures "d115" distance of L14 L20
  measures "d117" distance of L15 L23
  measures "d118" distance of L16 L22
  measures "d161" distance of L30 L33.end
extrude "Extrude15" cut sketch "Sketch12" against normal blind 0.2 text T0 T1 T2 T3 bodies 1
sketch "Sketch13" plane through (0, 0, -1.6) normal (0, 0, 1) x (-1, 0, 0)
  line L0 (-6, 10.5) -> (-6, 3)
  line L1 (-6, 3) -> (-16.75, 3)
  line L2 (-16.75, 3) -> (-16.75, -0.25)
  line L3 (-16.75, -0.25) -> (-71.19, -0.25)
  line L4 (-71.19, -0.25) -> (-71.19, 3)
  line L5 (-71.19, 3) -> (-85.19, 3)
  line L6 (-85.19, 3) -> (-85.19, 10.5)
  line L7 (-85.19, 10.5) -> (-90.19, 10.5)
  line L8 (-90.19, 10.5) -> (-90.19, 18.5)
  line L9 (-90.19, 18.5) -> (-85.19, 18.5)
  line L10 (-85.19, 18.5) -> (-85.19, 26)
  line L11 (-85.19, 26) -> (-71.69, 26)
  line L12 (-71.69, 26) -> (-71.69, 30)
  line L13 (-71.69, 30) -> (-61.19, 30)
  line L14 (-61.19, 30) -> (-61.19, 29.25)
  line L15 (-61.19, 29.25) -> (-6, 29.25)
  line L16 (-6, 29.25) -> (-6, 18.5)
  line L17 (-6, 18.5) -> (-1, 18.5)
  line L18 (-1, 18.5) -> (-1, 10.5)
  line L19 (-1, 10.5) -> (-6, 10.5)
  circle A0 centre (-1.97, 2) radius 1.4
  circle A1 centre (-1.97, 27) radius 1.4
  circle A2 centre (-89.22, 2) radius 1.4
  circle A3 centre (-89.22, 27) radius 1.4
  line L20 (-0.75, 31.25) -> (-90.44, 31.25)
  arc A4 (-90.44, 31.25) -> (-93.44, 28.25) centre (-90.44, 28.25) ccw
  line L21 (-93.44, 28.25) -> (-93.44, 0.75)
  arc A5 (-93.44, 0.75) -> (-90.44, -2.25) centre (-90.44, 0.75) ccw
  line L22 (-90.44, -2.25) -> (-0.75, -2.25)
  arc A6 (-0.75, -2.25) -> (2.25, 0.75) centre (-0.75, 0.75) ccw
  line L23 (2.25, 0.75) -> (2.25, 28.25)
  arc A7 (2.25, 28.25) -> (-0.75, 31.25) centre (-0.75, 28.25) ccw
  line L24 (-1.5, 10) -> (-1.5, 10.5)
  constraint coincident L19 L24.end
  constraint perpendicular L19 L24
extrude "Extrude16" cut sketch "Sketch13" against normal up to surface (3 mm away) contours L0 L1 L2 L3 L4 L5 L6 L7 L8 L9 L10 L11 L12 L13 L14 L15 L16 L17 L18 L19 bodies 2
sketch "Sketch14" plane through (0, 0, -22.6) normal (0, 0, -1) x (1, 0, 0)
  line L0 (90.44, 31.25) -> (0.75, 31.25)
  arc A0 (0.75, 31.25) -> (-2.25, 28.25) centre (0.75, 28.25) ccw
  line L1 (-2.25, 28.25) -> (-2.25, 0.75)
  arc A1 (-2.25, 0.75) -> (0.75, -2.25) centre (0.75, 0.75) ccw
  line L2 (0.75, -2.25) -> (90.44, -2.25)
  arc A2 (90.44, -2.25) -> (93.44, 0.75) centre (90.44, 0.75) ccw
  line L3 (93.44, 0.75) -> (93.44, 28.25)
  arc A3 (93.44, 28.25) -> (90.44, 31.25) centre (90.44, 28.25) ccw
  circle A4 centre (89.22, 27) radius 1.4
  circle A5 centre (1.97, 27) radius 1.4
  circle A6 centre (89.22, 2) radius 1.4
  circle A7 centre (1.97, 2) radius 1.4
  line L4 (6, 3) -> (6, 25)
  line L5 (6, 25) -> (61.19, 25)
  line L6 (61.19, 25) -> (61.19, 30)
  line L7 (61.19, 30) -> (71.69, 30)
  line L8 (71.69, 30) -> (71.69, 26)
  line L9 (71.69, 26) -> (85.19, 26)
  line L10 (85.19, 26) -> (85.19, 3)
  line L11 (85.19, 3) -> (6, 3)
  line L12 (56.1905, 23.2909) -> (60.507, 23.2909) construction
  line L13 (60.507, 23.2909) -> (60.507, 30.25) construction
  line L14 (60.507, 30.25) -> (56.1905, 30.25) construction
  line L15 (56.1905, 30.25) -> (56.1905, 23.2909) construction
  line L16 (72.69, 23.4065) -> (84.7618, 23.4065) construction
  line L17 (84.7618, 23.4065) -> (84.7618, 30.25) construction
  line L18 (84.7618, 30.25) -> (72.69, 30.25) construction
  line L19 (72.69, 30.25) -> (72.69, 23.4065) construction
  line L20 (-2.25, 14.5) -> (93.44, 14.5) construction
  line L21 (-0.75, 15.25) -> (4.25, 15.25)
  line L22 (4.25, 15.25) -> (4.25, 13.75)
  line L23 (4.25, 13.75) -> (-0.75, 13.75)
  line L24 (-0.75, 13.75) -> (-0.75, 15.25)
  line L25 (1, 17) -> (2.5, 17)
  line L26 (2.5, 17) -> (2.5, 12)
  line L27 (2.5, 12) -> (1, 12)
  line L28 (1, 12) -> (1, 17)
  line L29 (1.75, 17) -> (1.75, 12) construction
  line L30 (-0.75, 14.5) -> (4.25, 14.5)
  line L31 (88.565, 17) -> (90.065, 17)
  line L32 (90.065, 17) -> (90.065, 12)
  line L33 (90.065, 12) -> (88.565, 12)
  line L34 (88.565, 12) -> (88.565, 17)
  line L35 (89.315, 17) -> (89.315, 12) construction
  dimension "d119" = 6.25
  dimension "d120" = 1
  dimension "d121" = 1
  dimension "d122" = 4.3165
  dimension "d123" = 0.683
  dimension "d129" = 5
  dimension "d130" = 1.5
  dimension "d131" = 1.5
  dimension "d132" = 1.5
  dimension "d133" = 5
  text T0 "S" font "Arial" height 4 bold align left top in box 4.3165 x 6.9591 at (56.1905, 23.2909) x (1, 0) y (0, 1) spacing 1
  text T1 "N" font "Arial" height 4 bold align left top in box 12.0718 x 6.8435 at (72.69, 23.4065) x (1, 0) y (0, 1) spacing 1
  constraint collinear L14 L18
  constraint midpoint L1 L20.start
  constraint midpoint L3 L20.end
  constraint horizontal L21
  constraint vertical L22
  constraint horizontal L23
  constraint vertical L24
  constraint horizontal L25
  constraint vertical L26
  constraint horizontal L27
  constraint vertical L28
  constraint equal L24 L25
  constraint symmetric L20 L21 L23
  constraint midpoint L25 L29.start
  constraint midpoint L27 L29.end
  constraint midpoint L24 L30.start
  constraint midpoint L22 L30.end
  constraint midpoint L29 L30
  constraint equal L21 L28
  constraint horizontal L31
  constraint vertical L32
  constraint horizontal L33
  constraint vertical L34
  constraint symmetric L20 L31 L33
  constraint midpoint L31 L35.start
  constraint midpoint L33 L35.end
  measures "d119" distance of L0 L5
  measures "d120" distance of L0 L14
  measures "d121" distance of L8 L19
  measures "d123" distance of L6 L13
  measures "d129" distance of L21.start L21.end
  measures "d130" distance of L25.start L25.end
  measures "d131" distance of L1 L24
  measures "d132" distance of L31.start L31.end
  measures "d133" distance of L31.end L32.end
extrude "Extrude17" cut sketch "Sketch14" sketch "Sketch14" against normal blind 0.2 contours L21 L24 L28 L30 | L21 L25 L26 L28 | L21 L26 L28 L30 | L23 L24 L28 L30 | L21 L22 L26 L30 | L23 L26 L28 L30 | L22 L23 L26 L30 | L23 L26 L27 L28 | L31 L32 L33 L34 of sketch 2 text T0 T1 bodies 2
sketch "Sketch15" plane through (0, 0, -22.6) normal (0, 0, -1) x (1, 0, 0)
  line L0 (90.065, 17) -> (90.065, 12)
  line L1 (90.065, 12) -> (88.565, 12)
  line L2 (88.565, 12) -> (88.565, 17)
  line L3 (88.565, 17) -> (90.065, 17)
  spline S0 degree 3 poles (57.8412, 26.1791) (57.611, 26.1873) (57.1901, 26.2024) (56.8364, 26.4276) (56.6761, 26.5297) knots 0 0 0 0 0.067624 0.123634 0.123634 0.123634 0.123634
  spline S1 degree 3 poles (56.6761, 26.5297) (56.5536, 26.6663) (56.292, 26.958) (56.2257, 27.3455) (56.1905, 27.5515) knots 0 0 0 0 0.053943 0.115202 0.115202 0.115202 0.115202
  line L4 (56.1905, 27.5515) -> (56.9763, 27.6279)
  spline S2 degree 3 poles (56.9763, 27.6279) (57.0021, 27.5084) (57.0494, 27.2896) (57.1971, 27.1225) (57.2641, 27.0467) knots 0 0 0 0 0.035954 0.065825 0.065825 0.065825 0.065825
  spline S3 degree 3 poles (57.2641, 27.0467) (57.3465, 26.9927) (57.5236, 26.8765) (57.7359, 26.8665) (57.8494, 26.8612) knots 0 0 0 0 0.02903 0.062403 0.062403 0.062403 0.062403
  spline S4 degree 3 poles (57.8494, 26.8612) (57.9666, 26.8644) (58.1775, 26.8702) (58.3575, 26.9783) (58.4374, 27.0263) knots 0 0 0 0 0.034457 0.061988 0.061988 0.061988 0.061988
  spline S5 degree 3 poles (58.4374, 27.0263) (58.4951, 27.0818) (58.6055, 27.1883) (58.6256, 27.3399) (58.6352, 27.4123) knots 0 0 0 0 0.023254 0.044539 0.044539 0.044539 0.044539
  spline S6 degree 3 poles (58.6352, 27.4123) (58.6321, 27.4575) (58.626, 27.5455) (58.5763, 27.6183) (58.552, 27.6538) knots 0 0 0 0 0.013295 0.025956 0.025956 0.025956 0.025956
  spline S7 degree 3 poles (58.552, 27.6538) (58.5154, 27.6872) (58.4305, 27.7643) (58.3227, 27.8044) (58.2614, 27.8271) knots 0 0 0 0 0.014739 0.034108 0.034108 0.034108 0.034108
  spline S8 degree 3 poles (58.2614, 27.8271) (58.184, 27.8503) (57.9701, 27.9144) (57.7532, 27.9677) (57.6148, 28.0017) knots 0 0 0 0 0.02424 0.066991 0.066991 0.066991 0.066991
  spline S9 degree 3 poles (57.6148, 28.0017) (57.4253, 28.0498) (57.0991, 28.1327) (56.8203, 28.3192) (56.7034, 28.3973) knots 0 0 0 0 0.058092 0.099984 0.099984 0.099984 0.099984
  spline S10 degree 3 poles (56.7034, 28.3973) (56.596, 28.5125) (56.3836, 28.7401) (56.3511, 29.0494) (56.3351, 29.2023) knots 0 0 0 0 0.04588 0.090697 0.090697 0.090697 0.090697
  spline S11 degree 3 poles (56.3351, 29.2023) (56.3426, 29.3029) (56.3578, 29.5063) (56.4578, 29.6841) (56.5083, 29.7739) knots 0 0 0 0 0.029886 0.060385 0.060385 0.060385 0.060385
  spline S12 degree 3 poles (56.5083, 29.7739) (56.574, 29.8579) (56.7092, 30.031) (56.9063, 30.1288) (57.0077, 30.1791) knots 0 0 0 0 0.031562 0.065038 0.065038 0.065038 0.065038
  spline S13 degree 3 poles (57.0077, 30.1791) (57.1265, 30.2196) (57.3815, 30.3065) (57.651, 30.3141) (57.7948, 30.3182) knots 0 0 0 0 0.037465 0.080342 0.080342 0.080342 0.080342
  spline S14 degree 3 poles (57.7948, 30.3182) (58.0213, 30.3115) (58.4299, 30.2995) (58.7748, 30.0841) (58.9285, 29.9881) knots 0 0 0 0 0.06651 0.119965 0.119965 0.119965 0.119965
  spline S15 degree 3 poles (58.9285, 29.9881) (59.0404, 29.8666) (59.27, 29.6172) (59.3085, 29.2798) (59.3283, 29.1068) knots 0 0 0 0 0.048247 0.099032 0.099032 0.099032 0.099032
  line L5 (59.3283, 29.1068) -> (58.5206, 29.0713)
  spline S16 degree 3 poles (58.5206, 29.0713) (58.5017, 29.164) (58.4673, 29.3326) (58.3508, 29.4581) (58.2982, 29.5147) knots 0 0 0 0 0.027726 0.050455 0.050455 0.050455 0.050455
  spline S17 degree 3 poles (58.2982, 29.5147) (58.2288, 29.5539) (58.0708, 29.6431) (57.8887, 29.6474) (57.7867, 29.6497) knots 0 0 0 0 0.023601 0.053634 0.053634 0.053634 0.053634
  spline S18 degree 3 poles (57.7867, 29.6497) (57.6796, 29.6464) (57.4842, 29.6402) (57.313, 29.5472) (57.2355, 29.5051) knots 0 0 0 0 0.031585 0.057684 0.057684 0.057684 0.057684
  spline S19 degree 3 poles (57.2355, 29.5051) (57.1981, 29.4717) (57.1237, 29.4053) (57.1127, 29.3061) (57.1073, 29.2568) knots 0 0 0 0 0.014496 0.028843 0.028843 0.028843 0.028843
  spline S20 degree 3 poles (57.1073, 29.2568) (57.1128, 29.2108) (57.1243, 29.1159) (57.1923, 29.0486) (57.2273, 29.014) knots 0 0 0 0 0.013503 0.02781 0.02781 0.02781 0.02781
  spline S21 degree 3 poles (57.2273, 29.014) (57.3134, 28.9672) (57.5463, 28.8406) (57.8059, 28.7829) (57.9695, 28.7466) knots 0 0 0 0 0.029285 0.079208 0.079208 0.079208 0.079208
  spline S22 degree 3 poles (57.9695, 28.7466) (58.1423, 28.7051) (58.4411, 28.6334) (58.7225, 28.5105) (58.8412, 28.4587) knots 0 0 0 0 0.05318 0.09196 0.09196 0.09196 0.09196
  spline S23 degree 3 poles (58.8412, 28.4587) (58.9299, 28.4052) (59.1048, 28.2996) (59.2243, 28.1339) (59.2832, 28.0522) knots 0 0 0 0 0.030713 0.060609 0.060609 0.060609 0.060609
  spline S24 degree 3 poles (59.2832, 28.0522) (59.3298, 27.9578) (59.4286, 27.7573) (59.4379, 27.5335) (59.4429, 27.4151) knots 0 0 0 0 0.031207 0.066326 0.066326 0.066326 0.066326
  spline S25 degree 3 poles (59.4429, 27.4151) (59.4346, 27.3019) (59.418, 27.0733) (59.3076, 26.8725) (59.2519, 26.7711) knots 0 0 0 0 0.033629 0.067874 0.067874 0.067874 0.067874
  spline S26 degree 3 poles (59.2519, 26.7711) (59.1807, 26.6771) (59.0359, 26.4859) (58.8209, 26.3793) (58.7116, 26.325) knots 0 0 0 0 0.03487 0.070919 0.070919 0.070919 0.070919
  spline S27 degree 3 poles (58.7116, 26.325) (58.5819, 26.2825) (58.2995, 26.19) (58.0021, 26.1829) (57.8412, 26.1791) knots 0 0 0 0 0.040722 0.088678 0.088678 0.088678 0.088678
  line L6 (73.4403, 28.8585) -> (73.4403, 26.25)
  line L7 (73.4403, 26.25) -> (72.69, 26.25)
  line L8 (72.69, 26.25) -> (72.69, 30.25)
  line L9 (72.69, 30.25) -> (73.4758, 30.25)
  line L10 (73.4758, 30.25) -> (75.1129, 27.5788)
  line L11 (75.1129, 27.5788) -> (75.1129, 30.25)
  line L12 (75.1129, 30.25) -> (75.8633, 30.25)
  line L13 (75.8633, 30.25) -> (75.8633, 26.25)
  line L14 (75.8633, 26.25) -> (75.0529, 26.25)
  line L15 (75.0529, 26.25) -> (73.4403, 28.8585)
  line L16 (2.5, 13.75) -> (2.5, 12)
  line L17 (2.5, 12) -> (1, 12)
  line L18 (1, 12) -> (1, 13.75)
  line L19 (1, 13.75) -> (-0.75, 13.75)
  line L20 (-0.75, 13.75) -> (-0.75, 15.25)
  line L21 (-0.75, 15.25) -> (1, 15.25)
  line L22 (1, 15.25) -> (1, 17)
  line L23 (1, 17) -> (2.5, 17)
  line L24 (2.5, 17) -> (2.5, 15.25)
  line L25 (2.5, 15.25) -> (4.25, 15.25)
  line L26 (4.25, 15.25) -> (4.25, 13.75)
  line L27 (4.25, 13.75) -> (2.5, 13.75)
  line L28 (90.44, 31.25) -> (0.75, 31.25)
  arc A0 (0.75, 31.25) -> (-2.25, 28.25) centre (0.75, 28.25) ccw
  line L29 (-2.25, 28.25) -> (-2.25, 0.75)
  arc A1 (-2.25, 0.75) -> (0.75, -2.25) centre (0.75, 0.75) ccw
  line L30 (0.75, -2.25) -> (90.44, -2.25)
  arc A2 (90.44, -2.25) -> (93.44, 0.75) centre (90.44, 0.75) ccw
  line L31 (93.44, 0.75) -> (93.44, 28.25)
  arc A3 (93.44, 28.25) -> (90.44, 31.25) centre (90.44, 28.25) ccw
  circle A4 centre (1.97, 27) radius 1.4
  line L32 (61.19, 25) -> (61.19, 30)
  line L33 (61.19, 30) -> (71.69, 30)
  line L34 (71.69, 30) -> (71.69, 26)
  line L35 (71.69, 26) -> (85.19, 26)
  line L36 (85.19, 26) -> (85.19, 3)
  line L37 (85.19, 3) -> (6, 3)
  line L38 (6, 3) -> (6, 25)
  line L39 (6, 25) -> (61.19, 25)
  circle A5 centre (89.22, 27) radius 1.4
  circle A6 centre (89.22, 2) radius 1.4
  circle A7 centre (1.97, 2) radius 1.4
extrude "Extrude18" add sketch "Sketch15" against normal blind 5 contours A4 | A5 | A6 | A7 bodies 2
fillet "Fillet6" radius 1.5 13 edges at (6, -3, -12.1) (6, -25, -21.35) (85.19, -3, -12.1) (61.19, -25, -21.35) (71.69, -30, -12.1) (61.19, -30, -12.1) (6, -29.25, -10.85) (16.75, -3, -10.85) (16.75, 0.25, -10.85) (71.19, 0.25, -10.85) (71.19, -3, -10.85) (71.69, -26, -12.1) (85.19, -26, -12.1) on bodies 2
sketch "Sketch16" plane through (-2.25, 0, 0) normal (-1, 0, 0) x (0, -1, 0)
  line L0 (28.25, -1.6) -> (0.75, -1.6)
  line L1 (0.75, -1.6) -> (0.75, -22.6)
  line L2 (0.75, -22.6) -> (28.25, -22.6)
  line L3 (28.25, -22.6) -> (28.25, -1.6)
  line L4 (7, 3.5) -> (10, 3.5)
  line L5 (6, 1) -> (6, 2.5)
  line L6 (10, 0) -> (7, 0)
  line L7 (11, 2.5) -> (11, 1)
  line L8 (6, -3.2) -> (11, -3.2)
  line L9 (11, -3.2) -> (11, -6.7)
  line L10 (11, -6.7) -> (6, -6.7)
  line L11 (6, -6.7) -> (6, -3.2)
  line L12 (8.5, 3.5) -> (8.5, 0) construction
  line L13 (8.5, -3.2) -> (8.5, -6.7) construction
  constraint horizontal L8
  constraint vertical L9
  constraint horizontal L10
  constraint vertical L11
  constraint collinear L5 L11
  constraint collinear L7 L9
  constraint midpoint L4 L12.start
  constraint midpoint L6 L12.end
  constraint midpoint L8 L13.start
  constraint midpoint L10 L13.end
  constraint equal L12 L13
extrude "Extrude19" cut sketch "Sketch16" against normal blind 17 contours L8 L9 L10 L11 bodies 2
sketch "Sketch17" plane through (0, 0, -3.2) normal (0, 0, -1) x (1, 0, 0)
  line L0 (1, 10.5) -> (1, 11)
  line L1 (1, 11) -> (-2.25, 11)
  line L2 (-2.25, 11) -> (-2.25, 6)
  line L3 (-2.25, 6) -> (6, 6)
  line L4 (6, 6) -> (6, 10.5)
  line L5 (6, 10.5) -> (1, 10.5)
  line L6 (1, 10.5) -> (1, 6)
  constraint coincident L0.start L5.end
  constraint coincident L3 L6.end
  constraint perpendicular L3 L6
extrude "Extrude20" cut sketch "Sketch17" against normal blind 13.5 contours L3 L4 L5 L6 bodies 2
fillet "Fillet7" radius 1 4 edges at (1.875, -11, -6.7) (1.875, -6, -6.7) (-0.625, -6, -3.2) (-0.625, -11, -3.2) on bodies 2